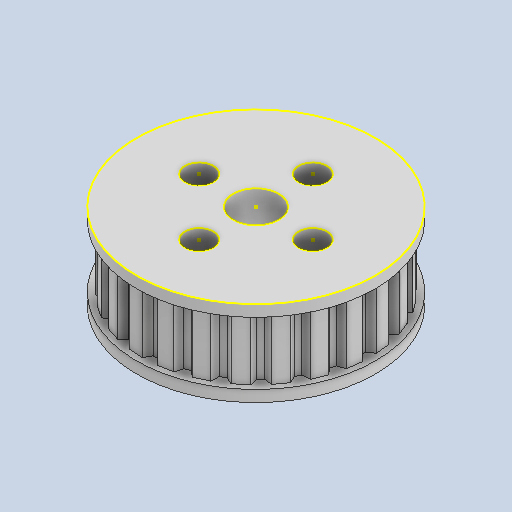
# Autodesk Inventor part: xl28 driven
Saved by Autodesk Inventor 2025 (Build 290162000, 162)
## iProperties
Created: 2025-04-12
Part Number: xl28 driven
Material: 一般
Document SubType Name: Modeling
Designer: gavin
Density: 1 g/cm^3
Appearance: 預設
Author: gavin
Autodesk Inventor part; units mm, degrees
ref_plane "YZ Plane" through (0, 0, 0) normal (1, 0, 0) x (0, 1, 0)
ref_plane "XZ Plane" through (0, 0, 0) normal (0, 1, 0) x (-1, 0, 0)
ref_plane "XY Plane" through (0, 0, 0) normal (0, 0, 1) x (1, 0, 0)
sketch "草圖1" plane through (0, 0, 0) normal (0, 1, 0) x (-1, 0, 0)
  line L0 (19.96, 1.2218) -> (19.96, -1.2218)
  line L1 (19.96, 0) -> (24.0887, 0) construction
  line L2 (18.69, 1.855) -> (19.96, 1.2218)
  line L3 (18.69, -1.855) -> (19.96, -1.2218)
  arc A0 (18.69, 1.855) -> (18.6093, 2.54) centre (0, 0) ccw
  arc A1 (18.6093, -2.54) -> (18.69, -1.855) centre (0, 0) ccw
  line L4 (19.0291, 6.1473) -> (19.6368, 3.7804)
  line L5 (17.6415, 6.4447) -> (19.0291, 6.1473)
  line L6 (18.5641, 2.8513) -> (19.6368, 3.7804)
  arc A2 (17.6415, 6.4447) -> (17.393, 7.0881) centre (0, 0) ccw
  arc A3 (18.6563, 2.1677) -> (18.5641, 2.8513) centre (0, 0) ccw
  line L7 (16.9025, 10.6865) -> (18.0797, 8.5451)
  line L8 (15.4845, 10.6295) -> (16.9025, 10.6865)
  line L9 (17.2718, 7.3784) -> (18.0797, 8.5451)
  arc A4 (15.4845, 10.6295) -> (15.0838, 11.1909) centre (0, 0) ccw
  arc A5 (17.5311, 6.7393) -> (17.2718, 7.3784) centre (0, 0) ccw
  line L10 (13.7138, 14.5542) -> (15.3866, 12.7729)
  line L11 (12.3546, 14.1464) -> (13.7138, 14.5542)
  line L12 (14.8943, 11.4419) -> (15.3866, 12.7729)
  arc A6 (12.3546, 14.1464) -> (11.8268, 14.5905) centre (0, 0) ccw
  arc A7 (15.3043, 10.8874) -> (14.8943, 11.4419) centre (0, 0) ccw
  line L13 (9.6635, 17.5075) -> (11.7267, 16.1981)
  line L14 (8.4484, 16.7744) -> (9.6635, 17.5075)
  line L15 (11.5808, 14.7865) -> (11.7267, 16.1981)
  arc A8 (8.4484, 16.7744) -> (7.8268, 17.0733) centre (0, 0) ccw
  arc A9 (12.1159, 14.3513) -> (11.5808, 14.7865) centre (0, 0) ccw
  line L16 (5.006, 19.3606) -> (7.33, 18.6055)
  line L17 (4.0113, 18.3485) -> (5.006, 19.3606)
  line L18 (7.5397, 17.202) -> (7.33, 18.6055)
  arc A10 (4.0113, 18.3485) -> (3.3349, 18.4834) centre (0, 0) ccw
  arc A11 (8.1663, 16.9136) -> (7.5397, 17.202) centre (0, 0) ccw
  line L19 (0.0339, 19.9973) -> (2.4727, 19.8439)
  line L20 (-0.6778, 18.7696) -> (0.0339, 19.9973)
  line L21 (3.0249, 18.5366) -> (2.4727, 19.8439)
  arc A12 (-0.6778, 18.7696) -> (-1.3665, 18.7321) centre (0, 0) ccw
  arc A13 (3.7035, 18.4131) -> (3.0249, 18.5366) centre (0, 0) ccw
  line L22 (-4.9403, 19.3775) -> (-2.54, 19.8354)
  line L23 (-5.3243, 18.0114) -> (-4.9403, 19.3775)
  line L24 (-1.68, 18.7065) -> (-2.54, 19.8354)
  arc A14 (-5.3243, 18.0114) -> (-5.982, 17.8037) centre (0, 0) ccw
  arc A15 (-0.992, 18.7556) -> (-1.68, 18.7065) centre (0, 0) ccw
  line L25 (-9.6041, 17.5401) -> (-7.393, 18.5806)
  line L26 (-9.6363, 16.1214) -> (-9.6041, 17.5401)
  line L27 (-6.2794, 17.701) -> (-7.393, 18.5806)
  arc A16 (-9.6363, 16.1214) -> (-10.2217, 15.7567) centre (0, 0) ccw
  arc A17 (-5.6252, 17.9197) -> (-6.2794, 17.701) centre (0, 0) ccw
  line L28 (-13.6644, 14.6006) -> (-11.7816, 16.1582)
  line L29 (-13.3428, 13.2185) -> (-13.6644, 14.6006)
  line L30 (-10.4842, 15.5833) -> (-11.7816, 16.1582)
  arc A18 (-13.3428, 13.2185) -> (-13.8191, 12.7196) centre (0, 0) ccw
  arc A19 (-9.9049, 15.9578) -> (-10.4842, 15.5833) centre (0, 0) ccw
  line L31 (-16.8661, 10.7437) -> (-15.4298, 12.7207)
  line L32 (-16.2109, 9.485) -> (-16.8661, 10.7437)
  line L33 (-14.0302, 12.4864) -> (-15.4298, 12.7207)
  arc A20 (-16.2109, 9.485) -> (-16.5482, 8.8834) centre (0, 0) ccw
  arc A21 (-13.5623, 12.9932) -> (-14.0302, 12.4864) centre (0, 0) ccw
  line L34 (-19.0081, 6.2118) -> (-18.1086, 8.4838)
  line L35 (-18.0604, 5.1555) -> (-19.0081, 6.2118)
  line L36 (-16.6947, 8.605) -> (-18.1086, 8.4838)
  arc A22 (-18.0604, 5.1555) -> (-18.2375, 4.4889) centre (0, 0) ccw
  arc A23 (-16.3674, 9.2122) -> (-16.6947, 8.605) centre (0, 0) ccw
  line L37 (-19.9557, 1.2895) -> (-19.6495, 3.7138)
  line L38 (-18.7751, 0.5021) -> (-19.9557, 1.2895)
  line L39 (-18.3101, 4.1829) -> (-19.6495, 3.7138)
  arc A24 (-18.7751, 0.5021) -> (-18.7809, -0.1876) centre (0, 0) ccw
  arc A25 (-18.1442, 4.8523) -> (-18.3101, 4.1829) centre (0, 0) ccw
  line L40 (-19.6495, -3.7138) -> (-19.9557, -1.2895)
  line L41 (-18.3101, -4.1829) -> (-19.6495, -3.7138)
  line L42 (-18.7751, -0.5021) -> (-19.9557, -1.2895)
  arc A26 (-18.3101, -4.1829) -> (-18.1442, -4.8523) centre (0, 0) ccw
  arc A27 (-18.7809, 0.1876) -> (-18.7751, -0.5021) centre (0, 0) ccw
  line L43 (-18.1086, -8.4838) -> (-19.0081, -6.2118)
  line L44 (-16.6947, -8.605) -> (-18.1086, -8.4838)
  line L45 (-18.0604, -5.1555) -> (-19.0081, -6.2118)
  arc A28 (-16.6947, -8.605) -> (-16.3674, -9.2122) centre (0, 0) ccw
  arc A29 (-18.2375, -4.4889) -> (-18.0604, -5.1555) centre (0, 0) ccw
  line L46 (-15.4298, -12.7207) -> (-16.8661, -10.7437)
  line L47 (-14.0302, -12.4864) -> (-15.4298, -12.7207)
  line L48 (-16.2109, -9.485) -> (-16.8661, -10.7437)
  arc A30 (-14.0302, -12.4864) -> (-13.5623, -12.9932) centre (0, 0) ccw
  arc A31 (-16.5482, -8.8834) -> (-16.2109, -9.485) centre (0, 0) ccw
  line L49 (-11.7816, -16.1582) -> (-13.6644, -14.6006)
  line L50 (-10.4842, -15.5833) -> (-11.7816, -16.1582)
  line L51 (-13.3428, -13.2185) -> (-13.6644, -14.6006)
  arc A32 (-10.4842, -15.5833) -> (-9.9049, -15.9578) centre (0, 0) ccw
  arc A33 (-13.8191, -12.7196) -> (-13.3428, -13.2185) centre (0, 0) ccw
  line L52 (-7.393, -18.5806) -> (-9.6041, -17.5401)
  line L53 (-6.2794, -17.701) -> (-7.393, -18.5806)
  line L54 (-9.6363, -16.1214) -> (-9.6041, -17.5401)
  arc A34 (-6.2794, -17.701) -> (-5.6252, -17.9197) centre (0, 0) ccw
  arc A35 (-10.2217, -15.7567) -> (-9.6363, -16.1214) centre (0, 0) ccw
  line L55 (-2.54, -19.8354) -> (-4.9403, -19.3775)
  line L56 (-1.68, -18.7065) -> (-2.54, -19.8354)
  line L57 (-5.3243, -18.0114) -> (-4.9403, -19.3775)
  arc A36 (-1.68, -18.7065) -> (-0.992, -18.7556) centre (0, 0) ccw
  arc A37 (-5.982, -17.8037) -> (-5.3243, -18.0114) centre (0, 0) ccw
  line L58 (2.4727, -19.8439) -> (0.0339, -19.9973)
  line L59 (3.0249, -18.5366) -> (2.4727, -19.8439)
  line L60 (-0.6778, -18.7696) -> (0.0339, -19.9973)
  arc A38 (3.0249, -18.5366) -> (3.7035, -18.4131) centre (0, 0) ccw
  arc A39 (-1.3665, -18.7321) -> (-0.6778, -18.7696) centre (0, 0) ccw
  line L61 (7.33, -18.6055) -> (5.006, -19.3606)
  line L62 (7.5397, -17.202) -> (7.33, -18.6055)
  line L63 (4.0113, -18.3485) -> (5.006, -19.3606)
  arc A40 (7.5397, -17.202) -> (8.1663, -16.9136) centre (0, 0) ccw
  arc A41 (3.3349, -18.4834) -> (4.0113, -18.3485) centre (0, 0) ccw
  line L64 (11.7267, -16.1981) -> (9.6635, -17.5075)
  line L65 (11.5808, -14.7865) -> (11.7267, -16.1981)
  line L66 (8.4484, -16.7744) -> (9.6635, -17.5075)
  arc A42 (11.5808, -14.7865) -> (12.1159, -14.3513) centre (0, 0) ccw
  arc A43 (7.8268, -17.0733) -> (8.4484, -16.7744) centre (0, 0) ccw
  line L67 (15.3866, -12.7729) -> (13.7138, -14.5542)
  line L68 (14.8943, -11.4419) -> (15.3866, -12.7729)
  line L69 (12.3546, -14.1464) -> (13.7138, -14.5542)
  arc A44 (14.8943, -11.4419) -> (15.3043, -10.8874) centre (0, 0) ccw
  arc A45 (11.8268, -14.5905) -> (12.3546, -14.1464) centre (0, 0) ccw
  line L70 (18.0797, -8.5451) -> (16.9025, -10.6865)
  line L71 (17.2718, -7.3784) -> (18.0797, -8.5451)
  line L72 (15.4845, -10.6295) -> (16.9025, -10.6865)
  arc A46 (17.2718, -7.3784) -> (17.5311, -6.7393) centre (0, 0) ccw
  arc A47 (15.0838, -11.1909) -> (15.4845, -10.6295) centre (0, 0) ccw
  line L73 (19.6368, -3.7804) -> (19.0291, -6.1473)
  line L74 (18.5641, -2.8513) -> (19.6368, -3.7804)
  line L75 (17.6415, -6.4447) -> (19.0291, -6.1473)
  arc A48 (18.5641, -2.8513) -> (18.6563, -2.1677) centre (0, 0) ccw
  arc A49 (17.393, -7.0881) -> (17.6415, -6.4447) centre (0, 0) ccw
  circle A50 centre (0, 0) radius 4
  point P0 (19.3329, 4.9639)
  point P1 (17.4911, 9.6158)
  point P2 (14.5502, 13.6636)
  point P3 (10.6951, 16.8528)
  point P4 (6.168, 18.9831)
  point P5 (1.2533, 19.9206)
  point P6 (-3.7401, 19.6065)
  point P7 (-8.4986, 18.0603)
  point P8 (-12.723, 15.3794)
  point P9 (-16.148, 11.7322)
  point P10 (-18.5583, 7.3478)
  point P11 (-19.8026, 2.5017)
  point P12 (-19.8026, -2.5017)
  point P13 (-18.5583, -7.3478)
  point P14 (-16.148, -11.7322)
  point P15 (-12.723, -15.3794)
  point P16 (-8.4986, -18.0603)
  point P17 (-3.7401, -19.6065)
  point P18 (1.2533, -19.9206)
  point P19 (6.168, -18.9831)
  point P20 (10.6951, -16.8528)
  point P21 (14.5502, -13.6636)
  point P22 (17.4911, -9.6158)
  point P23 (19.3329, -4.9639)
  point P24 (18.6093, 2.54)
  point P25 (17.393, 7.0881)
  point P26 (15.0838, 11.1909)
  point P27 (11.8268, 14.5905)
  point P28 (7.8268, 17.0733)
  point P29 (3.3349, 18.4834)
  point P30 (-1.3665, 18.7321)
  point P31 (-5.982, 17.8037)
  point P32 (-10.2217, 15.7567)
  point P33 (-13.8191, 12.7196)
  point P34 (-16.5482, 8.8834)
  point P35 (-18.2375, 4.4889)
  point P36 (-18.7809, -0.1876)
  point P37 (-18.1442, -4.8523)
  point P38 (-16.3674, -9.2122)
  point P39 (-13.5623, -12.9932)
  point P40 (-9.9049, -15.9578)
  point P41 (-5.6252, -17.9197)
  point P42 (-0.992, -18.7556)
  point P43 (3.7035, -18.4131)
  point P44 (8.1663, -16.9136)
  point P45 (12.1159, -14.3513)
  point P46 (15.3043, -10.8874)
  point P47 (17.5311, -6.7393)
  point P48 (18.6093, -2.54)
  dimension "d8" = 360
  dimension "d10" = 8
  constraints: 152 end point, 100 point on circle, 51 centre point, 25 midpoint, 2 coincident, 2 symmetric about line, 1 perpendicular, 1 vertical, 326 other
  measures "d10" diameter of A50
extrude "擠出1" add sketch "草圖1" along normal blind 11
sketch "草圖2" plane through (0, 11, 0) normal (0, 1, 0) x (1, 0, 0)
  circle A0 centre (0, 0) radius 21
  circle A1 centre (0, 0) radius 4 projected
  dimension "d13" = 42
  constraints: 1 centre point, 1 coincident
  measures "d13" diameter of A0
extrude "擠出2" add sketch "草圖2" along normal blind 2
sketch "草圖3" plane through (0, 0, 0) normal (0, -1, 0) x (1, 0, 0)
  circle A0 centre (0, 0) radius 21 projected
  circle A1 centre (0, 0) radius 4 projected
extrude "擠出3" add sketch "草圖3" along normal blind 2
sketch "草圖4" plane through (0, 13, 0) normal (0, 1, 0) x (1, 0, 0)
  circle A0 centre (0, 0) radius 4 projected
  circle A1 centre (0, 0) radius 10 construction
  circle A2 centre (10, 0) radius 2.5
  circle A3 centre (0, 10) radius 2.5
  circle A4 centre (-10, 0) radius 2.5
  circle A5 centre (0, -10) radius 2.5
  dimension "d18" = 20
  dimension "d19" = 5
  dimension "d22" = 360
  constraints: 4 centre point, 1 coincident, 1 horizontal alignment, 11 other
  measures "d19" diameter of A2
extrude "擠出4" cut sketch "草圖4" against normal through all contours A2 | A3 | A4 | A5
sketch "草圖6" plane through (0, 13, 0) normal (0, 1, 0) x (1, 0, 0)
  circle A0 centre (0, -10) radius 2.5 projected
  circle A1 centre (0, 10) radius 2.5 projected
  circle A2 centre (-10, 0) radius 2.5 projected
  circle A3 centre (10, 0) radius 2.5 projected
  circle A4 centre (0, 0) radius 21 projected
  circle A5 centre (0, 0) radius 4 projected
equation "\"d2\" = 0.5 * d1"
equation "\"d1\" = 5.08"
